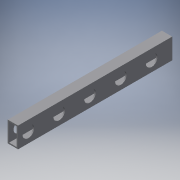
# Autodesk Inventor part: intake 1
Saved by Autodesk Inventor 2018.2 (Build 222227000, 227)
## iProperties
Created: 2018-02-02
Part Number: intake 1
Material: Generic
Document SubType Name: Modeling
Designer: Luke
Density: 1 g/cm^3
Appearance: Default
Author: Luke
Autodesk Inventor part; units mm, degrees
ref_plane "YZ Plane" through (0, 0, 0) normal (1, 0, 0) x (0, 1, 0)
ref_plane "XZ Plane" through (0, 0, 0) normal (0, 1, 0) x (-1, 0, 0)
ref_plane "XY Plane" through (0, 0, 0) normal (0, 0, 1) x (1, 0, 0)
sketch "Sketch1" plane through (0, 0, 0) normal (0, 0, 1) x (1, 0, 0)
  line L0 (0, 0) -> (25.4, 0)
  line L1 (25.4, 0) -> (25.4, -50.8)
  line L2 (25.4, -50.8) -> (0, -50.8)
  line L3 (0, -50.8) -> (0, 0)
  line L4 (22.225, -3.175) -> (3.175, -3.175)
  line L5 (3.175, -3.175) -> (3.175, -47.625)
  line L6 (3.175, -47.625) -> (22.225, -47.625)
  line L7 (22.225, -47.625) -> (22.225, -3.175)
  dimension "d0" = 25.4
  dimension "d1" = 50.8
  dimension "d2" = 3.175
  constraints: 16 end point, 4 parallel, 2 perpendicular, 1 horizontal, 3 other
  measures "d0" distance of L1.end L2.end
  measures "d1" distance of L0.end L1.end
  measures "d2" distance between parallel lines of L0 L4
extrude "Extrusion1" add sketch "Sketch1" along normal blind 381
sketch "Sketch2" plane through (25.4, -50.8, 0) normal (1, 0, 0) x (0, 0, -1)
  circle A0 centre (-355.6, 25.4) radius 14.2875
  circle A1 centre (-203.2, 25.4) radius 14.2875
  circle A2 centre (-50.8, 25.4) radius 14.2875
  line L0 (0, 0) -> (-381, 0) projected
  line L1 (0, 50.8) -> (-381, 50.8) projected
  line L2 (0, 50.8) -> (0, 0) projected
  dimension "d6" = 28.575
  dimension "d7" = 28.575
  dimension "d8" = 28.575
  dimension "d10" = 25.4
  dimension "d11" = 25.4
  dimension "d12" = 25.4
  dimension "d13" = 50.8
  dimension "d14" = 152.4
  dimension "d15" = 152.4
  constraints: 3 centre point
  measures "d6" diameter of A0
  measures "d7" diameter of A1
  measures "d8" diameter of A2
  measures "d10" distance from line of L1 A0.centre
  measures "d11" distance from line of L1 A1.centre
  measures "d12" distance from line of L0 A2.centre
  measures "d13" distance from line of L2 A2.centre
  measures "d14" distance of A2.centre A1.centre
  measures "d15" distance of A1.centre A0.centre
extrude "Extrusion2" cut sketch "Sketch2" against normal blind 381
sketch "Sketch3" plane through (0, -50.8, 0) normal (-1, 0, 0) x (0, 0, 1)
  circle A0 centre (127, 25.4) radius 14.2875
  circle A1 centre (279.4, 25.4) radius 14.2875
  line L0 (0, 0) -> (381, 0) projected
  circle A2 centre (203.2, 25.4) radius 14.2875 projected
  circle A3 centre (355.6, 25.4) radius 14.2875 projected
  point P0 (0, 50.8)
  dimension "d19" = 28.575
  dimension "d20" = 28.575
  dimension "d21" = 25.4
  dimension "d22" = 25.4
  dimension "d23" = 76.2
  dimension "d24" = 76.2
  dimension "d25" = 76.2
  constraints: 2 centre point
  measures "d19" diameter of A1
  measures "d20" diameter of A0
  measures "d21" distance from line of L0 A0.centre
  measures "d22" distance from line of L0 A1.centre
  measures "d23" distance of A2.centre A1.centre
  measures "d24" distance of A3.centre A1.centre
  measures "d25" distance of A2.centre A0.centre
extrude "Extrusion3" cut sketch "Sketch3" against normal blind 25.4 contours A0 | A1
body "Solid1"
